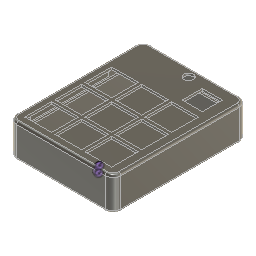
macropad (Autodesk Fusion 360 design; units mm, degrees)
part number: 2026-07-30-09-30-28-857
Autodesk Fusion 360 part; units mm, degrees
note: some values were not read from the file. Set by a fixed rule: which sketch regions a step uses.
(part 1 of 2)
sketch "Sketch1" plane through (0, 0, 0) normal (0, 0, 1) x (1, 0, 0)
  line L0 (0, 0) -> (61.8, 0)
  line L1 (61.8, 0) -> (61.8, 80.8)
  line L2 (61.8, 80.8) -> (0, 80.8)
  line L3 (0, 80.8) -> (0, 0)
  line L4 (-2.3, 78.1) -> (-2.3, 2.7)
  line L5 (2.7, -2.3) -> (59.1, -2.3)
  line L6 (64.1, 2.7) -> (64.1, 78.1)
  line L7 (59.1, 83.1) -> (2.7, 83.1)
  arc A0 (2.7, 83.1) -> (-2.3, 78.1) centre (2.7, 78.1) ccw
  arc A1 (64.1, 78.1) -> (59.1, 83.1) centre (59.1, 78.1) ccw
  arc A2 (59.1, -2.3) -> (64.1, 2.7) centre (59.1, 2.7) ccw
  arc A3 (-2.3, 2.7) -> (2.7, -2.3) centre (2.7, 2.7) ccw
  line L8 (60.5, 1.3) -> (60.5, 79.5)
  line L9 (60.5, 79.5) -> (1.3, 79.5)
  line L10 (1.3, 79.5) -> (1.3, 1.3)
  line L11 (1.3, 1.3) -> (60.5, 1.3)
  dimension "d1" = 61.8
  dimension "d2" = 80.8
  dimension "d4" = 5
  dimension "d5" = 5
  dimension "d6" = 5
  dimension "d7" = 5
  dimension "d17" = -1.3
  constraint horizontal L0
  constraint vertical L1
  constraint horizontal L2
  constraint vertical L3
  constraint coincident L0.start L3.end
  constraint tangent L4 A0
  constraint tangent L7 A0
  constraint tangent L6 A1
  constraint tangent L7 A1
  constraint tangent L5 A2
  constraint tangent L6 A2
  constraint tangent L4 A3
  constraint tangent L5 A3
  measures "d1" distance of L0.start L0.end
  measures "d2" distance of L0.start L2.end
  measures "d4" radius of A0
  measures "d5" radius of A1
  measures "d6" radius of A2
  measures "d7" radius of A3
extrude "Extrude1" add sketch "Sketch1" along normal blind 13.5 contours L0 L1 L2 L3 picked at (0.433333, 53.433333) makes body 1
extrude "Extrude2" add sketch "Sketch1" along normal blind 19.8 contours L4 L5 L6 L7 A0 A1 A2 A3 picked at (-0.766667, 52.966667) bodies 1
sketch "Sketch2" plane through (-2.3, 0, 0) normal (-1, 0, 0) x (0, -1, 0)
  line L0 (-78.1, 0) -> (-2.7, 0)
  line L1 (-2.7, 0) -> (-2.7, 19.8)
  line L2 (-2.7, 19.8) -> (-78.1, 19.8)
  line L3 (-78.1, 19.8) -> (-78.1, 0)
  line L4 (-74, 19.8) -> (-65, 19.8)
  line L5 (-65, 19.8) -> (-65, 16.2)
  line L6 (-65, 16.2) -> (-74, 16.2)
  line L7 (-74, 16.2) -> (-74, 19.8)
  line L8 (-78.1, 0) -> (-2.7, 0)
  point P0 (-80.8, 19.8)
  point P1 (-83.1, 19.8)
  dimension "d12" = 9
  dimension "d13" = 3.6
  dimension "d24" = 6.8
  constraint horizontal L4
  constraint vertical L5
  constraint horizontal L6
  constraint vertical L7
  constraint horizontal L4.start P1
  measures "d12" distance of L4.start L4.end
  measures "d13" distance of L4.start L6.end
  measures "d24" distance of L7 P0
extrude "Extrude3" add sketch "Sketch1" along normal blind 1.5 contours L8 L9 L10 L11 picked at (21.033333, 27.366667) bodies 1
extrude "Extrude4" cut sketch "Sketch2" against normal blind 13 contours L2 L4 L5 L6 L7 picked at (-71, 18.6) bodies 1
fillet "Fillet1" radius 0.5 2 edges at (-1.15, 74, 16.2) (-1.15, 65, 16.2) on bodies 1
sketch "Sketch4" plane through (0, 0, 0) normal (0, 0, 1) x (1, 0, 0)
  line L0 (97.7, 78.1) -> (97.7, 2.7)
  line L1 (100, 0) -> (161.8, 0)
  arc A0 (164.1, 78.1) -> (159.1, 83.1) centre (159.1, 78.1) ccw
  line L2 (161.8, 80.8) -> (100, 80.8)
  arc A1 (97.7, 2.7) -> (102.7, -2.3) centre (102.7, 2.7) ccw
  arc A2 (159.1, -2.3) -> (164.1, 2.7) centre (159.1, 2.7) ccw
  line L3 (102.7, -2.3) -> (159.1, -2.3)
  line L4 (164.1, 2.7) -> (164.1, 78.1)
  line L5 (161.8, 0) -> (161.8, 80.8)
  line L6 (100, 80.8) -> (100, 0)
  arc A3 (102.7, 83.1) -> (97.7, 78.1) centre (102.7, 78.1) ccw
  line L7 (159.1, 83.1) -> (102.7, 83.1)
  line L8 (160.4, 67.5) -> (162.4, 67.5)
  line L9 (162.4, 67.5) -> (162.4, 7.5)
  line L10 (162.4, 7.5) -> (160.4, 7.5)
  line L11 (160.4, 7.5) -> (160.4, 67.5)
  line L12 (161.8, 40.4) -> (175, 40.4) construction
  line L13 (100, 32.5) -> (87.946958, 32.5) construction
  line L14 (99.4, 57.5) -> (101.4, 57.5)
  line L15 (101.4, 57.5) -> (101.4, 7.5)
  line L16 (101.4, 7.5) -> (99.4, 7.5)
  line L17 (99.4, 7.5) -> (99.4, 57.5)
  line L18 (137.8, 79.4) -> (157.8, 79.4)
  line L19 (157.8, 79.4) -> (157.8, 81.4)
  line L20 (157.8, 81.4) -> (137.8, 81.4)
  line L21 (137.8, 81.4) -> (137.8, 79.4)
  line L22 (110.9, -0.6) -> (150.9, -0.6)
  line L23 (150.9, -0.6) -> (150.9, 1.4)
  line L24 (150.9, 1.4) -> (110.9, 1.4)
  line L25 (110.9, 1.4) -> (110.9, -0.6)
  line L26 (130.9, 0) -> (130.9, -7) construction
  point P0 (100, 0)
  dimension "d26" = 61.8
  dimension "d27" = 80.8
  dimension "d28" = 2.3
  dimension "d30" = 2.3
  dimension "d31" = 2.3
  dimension "d32" = 5
  dimension "d33" = 5
  dimension "d34" = 5
  dimension "d35" = 5
  dimension "d36" = 2
  dimension "d37" = 60
  dimension "d38" = 1.4
  dimension "d39" = 32.5
  dimension "d40" = 2
  dimension "d41" = 50
  dimension "d42" = 1.4
  dimension "d123" = 20
  dimension "d124" = 2
  dimension "d125" = 1.4
  dimension "d126" = 40
  dimension "d127" = 2
  dimension "d128" = 1.4
  dimension "d131" = 4
  dimension "d153" = 2.3
  constraint horizontal L1
  constraint vertical L5
  constraint horizontal L2
  constraint vertical L6
  constraint coincident P0 L1.start
  constraint tangent L0 A3
  constraint tangent A3 L7
  constraint tangent A0 L4
  constraint tangent A0 L7
  constraint tangent A2 L3
  constraint tangent A2 L4
  constraint tangent L0 A1
  constraint tangent A1 L3
  constraint horizontal L8
  constraint vertical L9
  constraint horizontal L10
  constraint vertical L11
  constraint midpoint L5 L12.start
  constraint perpendicular L4 L12
  constraint coincident L6 L13.start
  constraint perpendicular L6 L13
  constraint horizontal L14
  constraint vertical L15
  constraint horizontal L16
  constraint vertical L17
  constraint symmetric L13 L14 L16
  constraint horizontal L10.end L15.end
  constraint horizontal L18
  constraint vertical L19
  constraint horizontal L20
  constraint vertical L21
  constraint horizontal L22
  constraint vertical L23
  constraint horizontal L24
  constraint vertical L25
  constraint midpoint L1 L26.start
  constraint perpendicular L3 L26
  constraint symmetric L23 L25 L26
  measures "d26" distance of P0 L1.end
  measures "d27" distance of L2.end P0
  measures "d28" distance of L0 L6
  measures "d30" distance of L4 L5
  measures "d31" distance of L2 L7
  measures "d32" radius of A3
  measures "d33" radius of A0
  measures "d34" radius of A2
  measures "d35" radius of A1
  measures "d36" distance of L8.start L8.end
  measures "d37" distance of L8.start L10.end
  measures "d38" distance of L5 L11
  measures "d39" distance of L1 L13
  measures "d40" distance of L14.start L14.end
  measures "d41" distance of L14.start L16.end
  measures "d42" distance of L6 L15
  measures "d123" distance of L18.start L18.end
  measures "d124" distance of L18.start L20.end
  measures "d125" distance of L2 L18
  measures "d126" distance of L22.start L22.end
  measures "d127" distance of L22.start L24.end
  measures "d128" distance of L1 L24
  measures "d131" distance of L5 L19
  measures "d153" distance of L1 L3
extrude "Extrude5" add sketch "Sketch4" against normal blind 1.5 separate body contours L0 A0 A1 A2 L3 L4 A3 L7 | L1 L2 L5 L6 L8 L10 L11 L14 L15 L16 L18 L19 L21 L23 L24 L25 | L1 L23 L24 L25 | L1 L22 L23 L25 | L6 L14 L16 L17 | L6 L14 L15 L16 | L5 L8 L10 L11 | L5 L8 L9 L10 | L2 L19 L20 L21 | L2 L18 L19 L21 picked at (113.5, 81.566667) picked at (140.733333, 44.166667) picked at (124.233333, 0.933333) picked at (124.233333, -0.4) picked at (99.6, 40.833333) picked at (100.466667, 24.166667) picked at (161.333333, 27.5) picked at (162, 47.5) picked at (144.466667, 81.2) picked at (144.466667, 79.866667) makes body 2
extrude "Extrude6" add sketch "Sketch4" against normal blind 5.5 contours L1 L23 L24 L25 | L1 L22 L23 L25 | L6 L14 L16 L17 | L6 L14 L15 L16 | L5 L8 L10 L11 | L5 L8 L9 L10 | L2 L19 L20 L21 | L2 L18 L19 L21 picked at (124.233333, 0.933333) picked at (124.233333, -0.4) picked at (99.6, 40.833333) picked at (100.466667, 24.166667) picked at (161.333333, 27.5) picked at (162, 47.5) picked at (144.466667, 81.2) picked at (144.466667, 79.866667) bodies 2
sketch "Sketch5" plane through (0, 7.5, 0) normal (0, -1, 0) x (1, 0, 0)
  line L0 (101.4, -1.5) -> (99.4, -1.5)
  line L1 (99.4, -1.5) -> (99.4, -5.5)
  line L2 (99.4, -5.5) -> (101.4, -5.5)
  line L3 (101.40018, -1.5) -> (101.90018, -1.500023)
  line L4 (101.4, -5.5) -> (101.90018, -1.500023)
  line L5 (101.40018, -1.5) -> (99.4, -1.5)
  line L6 (99.4, -5.5) -> (99.4, -1.5)
  line L7 (99.4, -5.5) -> (101.4, -5.5)
  line L8 (100.599998, -1.5) -> (100.599998, -5.5)
  line L9 (100.599998, -5.5) -> (99.6, -3.447432)
  line L10 (99.6, -3.447432) -> (100.599998, -1.5)
  line L11 (159.1, -1.5) -> (102.7, -1.5) construction
  line L12 (130.9, -1.5) -> (130.9, -4) construction
  line L13 (160.39982, -1.5) -> (162.4, -1.5)
  line L14 (160.4, -1.5) -> (162.4, -1.5)
  line L15 (162.4, -5.5) -> (162.4, -1.5)
  line L16 (161.200002, -5.5) -> (162.2, -3.447432)
  line L17 (162.2, -3.447432) -> (161.200002, -1.5)
  line L18 (160.4, -5.5) -> (159.89982, -1.500023)
  line L19 (162.4, -5.5) -> (160.4, -5.5)
  line L20 (160.39982, -1.5) -> (159.89982, -1.500023)
  line L21 (161.200002, -1.5) -> (161.200002, -5.5)
  line L22 (162.4, -5.5) -> (160.4, -5.5)
  line L23 (162.4, -1.5) -> (162.4, -5.5)
  point P0 (102.8, -1.5)
  point P1 (159.1, -1.5)
  point P2 (159, -1.5)
  dimension "d58" = 0.5
  dimension "d65" = 0.2
  dimension "d66" = 1
  constraint coincident L2.end L4.start
  constraint coincident L0.end L1.start
  constraint perpendicular L1 L5
  constraint coincident L1.end L2.start
  constraint perpendicular L7 L8
  constraint midpoint L11 L12.start
  constraint perpendicular L11 L12
  constraint symmetric L0.start L12 L14.start
  constraint symmetric L0.end L12 L13.end
  constraint symmetric L1.end L12 L15.start
  constraint symmetric L2.end L12 L18.start
  constraint symmetric P0 L12 P2
  constraint symmetric L11.end L12 P1
extrude "Extrude7" cut sketch "Sketch5" against normal blind 69 contours L0 L1 L2 L5 L6 L7 L9 L10 | L13 L14 L15 L16 L17 L19 L22 L23 picked at (99.866666, -4.815811) picked at (161.933334, -4.815811) bodies 2
extrude "Extrude8" add sketch "Sketch5" against normal blind 50 contours L0 L2 L3 L4 L5 L7 L8 picked at (100.866665, -2.833333) bodies 2
extrude "Extrude9" add sketch "Sketch5" against normal blind 60 contours L13 L14 L18 L19 L20 L21 L22 picked at (160.666607, -2.833333) bodies 2
sketch "Sketch8" plane through (150.9, 0, 0) normal (1, 0, 0) x (0, 1, 0)
  line L0 (1.4, -1.5) -> (-0.6, -1.5)
  line L1 (-0.6, -1.5) -> (-0.6, -5.5)
  line L2 (-0.6, -5.5) -> (1.4, -5.5)
  line L3 (1.4, -5.5) -> (1.4, -1.5)
  line L4 (1.40018, -1.5) -> (-0.6, -1.5)
  line L5 (1.4, -1.5) -> (-0.6, -1.5)
  line L6 (-0.6, -5.5) -> (1.4, -5.5)
  line L7 (-0.4, -3.447432) -> (0.599998, -1.5)
  line L8 (0.599998, -5.5) -> (-0.4, -3.447432)
  line L9 (-0.6, -1.5) -> (-0.6, -5.5)
  line L10 (0.599998, -1.5) -> (0.599998, -5.5)
  line L11 (-0.6, -5.5) -> (-0.6, -1.5)
  line L12 (1.40018, -1.5) -> (1.90018, -1.500023)
  line L13 (1.4, -5.5) -> (1.90018, -1.500023)
  line L14 (-0.6, -5.5) -> (1.4, -5.5)
  line L15 (78.1, -1.5) -> (2.7, -1.5) construction
  line L16 (40.4, -1.5) -> (40.4, -9) construction
  line L17 (81.4, -5.5) -> (79.4, -5.5)
  line L18 (81.2, -3.447432) -> (80.200002, -1.5)
  line L19 (79.4, -1.5) -> (81.4, -1.5)
  line L20 (79.39982, -1.5) -> (78.89982, -1.500023)
  line L21 (81.4, -5.5) -> (81.4, -1.5)
  line L22 (81.4, -5.5) -> (79.4, -5.5)
  line L23 (79.39982, -1.5) -> (81.4, -1.5)
  line L24 (81.4, -1.5) -> (81.4, -5.5)
  line L25 (79.4, -5.5) -> (79.4, -1.5)
  line L26 (80.200002, -5.5) -> (81.2, -3.447432)
  line L27 (81.4, -1.5) -> (81.4, -5.5)
  line L28 (79.4, -5.5) -> (78.89982, -1.500023)
  line L29 (80.200002, -1.5) -> (80.200002, -5.5)
  line L30 (79.4, -1.5) -> (81.4, -1.5)
  line L31 (81.4, -5.5) -> (79.4, -5.5)
  point P0 (2.8, -1.5)
  dimension "d132" = 0.5
  dimension "d133" = 0.2
  dimension "d134" = 1
  constraint coincident L2.end L3.start
  constraint coincident L0.end L1.start
  constraint perpendicular L4 L9
  constraint coincident L1.end L2.start
  constraint perpendicular L6 L10
  constraint midpoint L15 L16.start
  constraint perpendicular L15 L16
  constraint symmetric L0.start L16 L19.start
  constraint symmetric L0.end L16 L19.end
  constraint symmetric L1.end L16 L17.start
  constraint symmetric L2.end L16 L17.end
extrude "Extrude13" cut sketch "Sketch8" along normal blind 13 and the other way blind 46.5 contours L0 L1 L2 L4 L5 L6 L7 L8 L9 L11 L14 | L17 L18 L19 L21 L22 L23 L24 L26 L27 L30 L31 picked at (-0.133334, -4.815811) picked at (80.933334, -4.815811) bodies 2
extrude "Extrude14" add sketch "Sketch8" against normal blind 40 contours L3 L12 L13 picked at (1.566727, -2.833341) bodies 2
extrude "Extrude15" add sketch "Sketch8" along normal blind 6.9 and the other way blind 13.1 contours L20 L25 L28 picked at (79.233273, -2.833341) bodies 2
move_body "Move1" bodies 2 to x (1, 0, 0) y (0, 1, 0) z (0, 0, 1) at (-100, 0, 21.3)
ref_plane "WorkPlane1" through (30.9, 7.7, 9.9) normal (0, -1, 0) x (1, 0, 0)
sketch "Sketch6" plane through (0, 7.7, 0) normal (0, -1, 0) x (-1, 0, 0)
  line L0 (-0.599998, -15.8) -> (-1.4, -15.8)
  line L1 (-1.40018, -19.8) -> (-0.599998, -19.8)
  line L2 (-61.200002, -19.8) -> (-60.39982, -19.8)
  line L3 (-60.4, -15.8) -> (-61.200002, -15.8)
  line L4 (-0.599998, -19.8) -> (0.4, -17.852568)
  line L5 (0.4, -17.852568) -> (-0.599998, -15.8)
  line L6 (-1.4, -15.8) -> (-1.90018, -19.799977)
  line L7 (-1.90018, -19.799977) -> (-1.40018, -19.8)
  line L8 (-60.39982, -19.8) -> (-59.89982, -19.799977)
  line L9 (-59.89982, -19.799977) -> (-60.4, -15.8)
  line L10 (-61.200002, -15.8) -> (-62.2, -17.852568)
  line L11 (-62.2, -17.852568) -> (-61.200002, -19.8)
extrude "Extrude10" cut sketch "Sketch6" against normal blind 50 contours L0 L1 L4 L5 L6 L7 picked at (-0.80006, -17.817523) bodies 1
extrude "Extrude11" cut sketch "Sketch6" against normal blind 60 contours L2 L3 L8 L9 L10 L11 picked at (-60.99994, -17.817523) bodies 1
sketch "Sketch7" plane through (0, 0, 21.3) normal (0, 0, 1) x (-1, 0, 0)
  line L0 (-59.1, -83.1) -> (-2.7, -83.1)
  arc A0 (-2.7, -83.1) -> (2.3, -78.1) centre (-2.7, -78.1) ccw
  line L1 (2.3, -78.1) -> (2.3, -2.7)
  arc A1 (2.3, -2.7) -> (-2.7, 2.3) centre (-2.7, -2.7) ccw
  line L2 (-2.7, 2.3) -> (-59.1, 2.3)
  arc A2 (-59.1, 2.3) -> (-64.1, -2.7) centre (-59.1, -2.7) ccw
  line L3 (-64.1, -2.7) -> (-64.1, -78.1)
  arc A3 (-64.1, -78.1) -> (-59.1, -83.1) centre (-59.1, -78.1) ccw
  circle A4 centre (-49.8, -68.8) radius 4
  line L4 (-43.8, -74.8) -> (-55.8, -74.8)
  line L5 (-55.8, -74.8) -> (-55.8, -62.8)
  line L6 (-55.8, -62.8) -> (-43.8, -62.8)
  line L7 (-43.8, -62.8) -> (-43.8, -74.8)
  line L8 (2.3, -74) -> (0, -74)
  line L9 (0, -74) -> (0, -80.8)
  line L10 (0, -80.8) -> (-61.8, -80.8)
  line L11 (-61.8, -80.8) -> (-61.8, 0)
  line L12 (-61.8, 0) -> (0, 0)
  line L13 (0, 0) -> (0, -65)
  line L14 (0, -65) -> (2.3, -65)
  line L15 (2.3, -65) -> (2.3, -2.7)
  arc A5 (2.3, -2.7) -> (-2.7, 2.3) centre (-2.7, -2.7) ccw
  line L16 (-2.7, 2.3) -> (-59.1, 2.3)
  arc A6 (-59.1, 2.3) -> (-64.1, -2.7) centre (-59.1, -2.7) ccw
  line L17 (-64.1, -2.7) -> (-64.1, -78.1)
  arc A7 (-64.1, -78.1) -> (-59.1, -83.1) centre (-59.1, -78.1) ccw
  line L18 (-59.1, -83.1) -> (-2.7, -83.1)
  arc A8 (-2.7, -83.1) -> (2.3, -78.1) centre (-2.7, -78.1) ccw
  line L19 (2.3, -78.1) -> (2.3, -74)
  circle A9 centre (-32.7, -77.3) radius 3
  line L20 (-3.4, -19.3) -> (-19, -19.3)
  line L21 (-19, -19.3) -> (-19, -3.7)
  line L22 (-19, -3.7) -> (-3.4, -3.7)
  line L23 (-3.4, -3.7) -> (-3.4, -19.3)
  line L24 (-22.5, -19.3) -> (-38.1, -19.3)
  line L25 (-38.1, -19.3) -> (-38.1, -3.7)
  line L26 (-38.1, -3.7) -> (-22.5, -3.7)
  line L27 (-22.5, -3.7) -> (-22.5, -19.3)
  line L28 (-41.6, -19.3) -> (-57.2, -19.3)
  line L29 (-57.2, -19.3) -> (-57.2, -3.7)
  line L30 (-57.2, -3.7) -> (-41.6, -3.7)
  line L31 (-41.6, -3.7) -> (-41.6, -19.3)
  line L32 (-3.4, -38.4) -> (-19, -38.4)
  line L33 (-19, -38.4) -> (-19, -22.8)
  line L34 (-19, -22.8) -> (-3.4, -22.8)
  line L35 (-3.4, -22.8) -> (-3.4, -38.4)
  line L36 (-22.5, -41.9) -> (-22.5, -57.5)
  line L37 (-38.1, -41.9) -> (-22.5, -41.9)
  line L38 (-38.1, -57.5) -> (-38.1, -41.9)
  line L39 (-22.5, -57.5) -> (-38.1, -57.5)
  line L40 (-3.4, -41.9) -> (-3.4, -57.5)
  line L41 (-19, -41.9) -> (-3.4, -41.9)
  line L42 (-19, -57.5) -> (-19, -41.9)
  line L43 (-3.4, -57.5) -> (-19, -57.5)
  line L44 (-22.5, -22.8) -> (-22.5, -38.4)
  line L45 (-38.1, -22.8) -> (-22.5, -22.8)
  line L46 (-38.1, -38.4) -> (-38.1, -22.8)
  line L47 (-22.5, -38.4) -> (-38.1, -38.4)
  line L48 (-41.6, -22.8) -> (-41.6, -38.4)
  line L49 (-57.2, -22.8) -> (-41.6, -22.8)
  line L50 (-57.2, -38.4) -> (-57.2, -22.8)
  line L51 (-41.6, -38.4) -> (-57.2, -38.4)
  line L52 (-41.6, -41.9) -> (-41.6, -57.5)
  line L53 (-57.2, -41.9) -> (-41.6, -41.9)
  line L54 (-57.2, -57.5) -> (-57.2, -41.9)
  line L55 (-41.6, -57.5) -> (-57.2, -57.5)
  line L56 (-19.7, -41.2) -> (-2.7, -41.2)
  line L57 (-2.7, -41.2) -> (-2.7, -58.2)
  line L58 (-2.7, -58.2) -> (-19.7, -58.2)
  line L59 (-19.7, -58.2) -> (-19.7, -41.2)
  line L60 (-38.8, -41.2) -> (-21.8, -41.2)
  line L61 (-21.8, -41.2) -> (-21.8, -58.2)
  line L62 (-21.8, -58.2) -> (-38.8, -58.2)
  line L63 (-38.8, -58.2) -> (-38.8, -41.2)
  line L64 (-57.9, -41.2) -> (-40.9, -41.2)
  line L65 (-40.9, -41.2) -> (-40.9, -58.2)
  line L66 (-40.9, -58.2) -> (-57.9, -58.2)
  line L67 (-57.9, -58.2) -> (-57.9, -41.2)
  line L68 (-19.7, -22.1) -> (-2.7, -22.1)
  line L69 (-2.7, -22.1) -> (-2.7, -39.1)
  line L70 (-2.7, -39.1) -> (-19.7, -39.1)
  line L71 (-19.7, -39.1) -> (-19.7, -22.1)
  line L72 (-38.8, -22.1) -> (-21.8, -22.1)
  line L73 (-21.8, -22.1) -> (-21.8, -39.1)
  line L74 (-21.8, -39.1) -> (-38.8, -39.1)
  line L75 (-38.8, -39.1) -> (-38.8, -22.1)
  line L76 (-57.9, -22.1) -> (-40.9, -22.1)
  line L77 (-40.9, -22.1) -> (-40.9, -39.1)
  line L78 (-40.9, -39.1) -> (-57.9, -39.1)
  line L79 (-57.9, -39.1) -> (-57.9, -22.1)
  line L80 (-19.7, -3) -> (-2.7, -3)
  line L81 (-2.7, -3) -> (-2.7, -20)
  line L82 (-2.7, -20) -> (-19.7, -20)
  line L83 (-19.7, -20) -> (-19.7, -3)
  line L84 (-38.8, -3) -> (-21.8, -3)
  line L85 (-21.8, -3) -> (-21.8, -20)
  line L86 (-21.8, -20) -> (-38.8, -20)
  line L87 (-38.8, -20) -> (-38.8, -3)
  line L88 (-57.9, -3) -> (-40.9, -3)
  line L89 (-40.9, -3) -> (-40.9, -20)
  line L90 (-40.9, -20) -> (-57.9, -20)
  line L91 (-57.9, -20) -> (-57.9, -3)
  line L92 (-56.2, -75.2) -> (-56.2, -62.4)
  line L93 (-56.2, -62.4) -> (-43.4, -62.4)
  line L94 (-43.4, -62.4) -> (-43.4, -75.2)
  line L95 (-43.4, -75.2) -> (-56.2, -75.2)
  dimension "d70" = 8
  dimension "d73" = 12
  dimension "d74" = 12
  dimension "d75" = 6
  dimension "d76" = 6
  dimension "d79" = 6
  dimension "d80" = 6
  dimension "d81" = 6
  dimension "d83" = 35
  dimension "d84" = 5.8
  dimension "d85" = 15.6
  dimension "d86" = 15.6
  dimension "d87" = 3.7
  dimension "d88" = 3.4
  dimension "d89" = 15.6
  dimension "d90" = 15.6
  dimension "d91" = 3.5
  dimension "d92" = 15.6
  dimension "d93" = 15.6
  dimension "d94" = 3.5
  dimension "d95" = 15.6
  dimension "d96" = 15.6
  dimension "d97" = 15.6
  dimension "d98" = 15.6
  dimension "d99" = 15.6
  dimension "d100" = 15.6
  dimension "d101" = 15.6
  dimension "d102" = 15.6
  dimension "d103" = 15.6
  dimension "d104" = 15.6
  dimension "d105" = 15.6
  dimension "d106" = 15.6
  dimension "d107" = 3.5
  dimension "d108" = 3.5
  dimension "d109" = -0.7
  dimension "d110" = -0.7
  dimension "d111" = -0.7
  dimension "d112" = -0.7
  dimension "d113" = -0.7
  dimension "d114" = -0.7
  dimension "d115" = -0.7
  dimension "d116" = -0.7
  dimension "d117" = -0.7
  dimension "d121" = -0.4
  constraint horizontal L4
  constraint vertical L5
  constraint horizontal L6
  constraint vertical L7
  constraint horizontal L20
  constraint vertical L21
  constraint horizontal L22
  constraint vertical L23
  constraint horizontal L24
  constraint vertical L25
  constraint horizontal L26
  constraint vertical L27
  constraint horizontal L20.end L24.start
  constraint horizontal L28
  constraint vertical L29
  constraint horizontal L30
  constraint vertical L31
  constraint horizontal L24.end L28.start
  constraint horizontal L32
  constraint perpendicular L32 L33
  constraint perpendicular L33 L34
  constraint perpendicular L32 L35
  constraint horizontal L39
  constraint perpendicular L38 L39
  constraint perpendicular L37 L38
  constraint perpendicular L36 L39
  constraint horizontal L43
  constraint perpendicular L42 L43
  constraint perpendicular L41 L42
  constraint perpendicular L40 L43
  constraint horizontal L47
  constraint perpendicular L46 L47
  constraint perpendicular L45 L46
  constraint perpendicular L44 L47
  constraint horizontal L51
  constraint perpendicular L50 L51
  constraint perpendicular L49 L50
  constraint perpendicular L48 L51
  constraint horizontal L55
  constraint perpendicular L54 L55
  constraint perpendicular L53 L54
  constraint perpendicular L52 L55
  constraint vertical L20.start L34.end
  constraint vertical L32.start L40.start
  constraint horizontal L36.end L42.start
  constraint vertical L24.start L36.end
  constraint horizontal L32.end L44.end
  constraint vertical L24.start L44.end
  constraint horizontal L38.start L52.end
  constraint vertical L28.start L52.end
  constraint horizontal L46.start L48.end
  constraint vertical L28.start L48.end
  measures "d70" diameter of A4
  measures "d73" distance of L4.start L4.end
  measures "d74" distance of L4.start L6.end
  measures "d75" distance of A4.centre L4
  measures "d76" distance of A4.centre L5
  measures "d79" distance of L4 L10
  measures "d80" distance of L5 L11
  measures "d81" diameter of A9
  measures "d83" distance of L19 A9.centre
  measures "d84" distance of L18 A9.centre
  measures "d85" distance of L20.start L20.end
  measures "d86" distance of L20.start L22.end
  measures "d87" distance of L12 L22
  measures "d88" distance of L13 L23
  measures "d89" distance of L24.start L24.end
  measures "d90" distance of L24.start L26.end
  measures "d91" distance of L21 L27
  measures "d92" distance of L28.start L28.end
  measures "d93" distance of L28.start L30.end
  measures "d94" distance of L25 L31
  measures "d95" distance of L32.start L32.end
  measures "d96" distance of L32 L34
  measures "d97" distance of L36.end L38.start
  measures "d98" distance of L37 L39
  measures "d99" distance of L40.end L42.start
  measures "d100" distance of L41 L43
  measures "d101" distance of L44.end L46.start
  measures "d102" distance of L45 L47
  measures "d103" distance of L48.end L50.start
  measures "d104" distance of L49 L51
  measures "d105" distance of L52.end L54.start
  measures "d106" distance of L53 L55
  measures "d107" distance of L20 L34
  measures "d108" distance of L32 L41
extrude "Extrude12" cut sketch "Sketch7" against normal blind 9 contours A4 | L4 L5 L6 L7 | A9 | L20 L21 L22 L23 | L24 L25 L26 L27 | L28 L29 L30 L31 | L32 L33 L34 L35 | L36 L37 L38 L39 | L40 L41 L42 L43 | L44 L45 L46 L47 | L48 L49 L50 L51 | L52 L53 L54 L55 | L56 L57 L58 L59 | L60 L61 L62 L63 | L64 L65 L66 L67 | L68 L69 L70 L71 | L72 L73 L74 L75 | L76 L77 L78 L79 | L80 L81 L82 L83 | L84 L85 L86 L87 | L88 L89 L90 L91 | L92 L93 L94 L95 picked at (-49.312879, -70.438611) picked at (-49.70036, -74.129605) picked at (-31.013745, -77.005245) picked at (-13.8, -14.1) picked at (-27.7, -14.1) picked at (-46.8, -8.9) picked at (-8.6, -33.2) picked at (-32.9, -47.1) picked at (-8.6, -52.3) picked at (-32.9, -28) picked at (-52, -28) picked at (-52, -47.1) picked at (-13.8, -57.966667) picked at (-38.566667, -52.3) picked at (-52, -41.433333) picked at (-8.6, -38.866667) picked at (-27.7, -38.866667) picked at (-57.666667, -33.2) picked at (-8.6, -19.766667) picked at (-27.7, -19.766667) picked at (-41.133333, -14.1) picked at (-56.066667, -66.8) bodies 2
ref_plane "WorkPlane2" through (51.7, 40.4, 9.9) normal (1, 0, 0) x (0, 1, 0)
sketch "Sketch9" plane through (51.7, 0, 0) normal (1, 0, 0) x (0, 1, 0)
  line L0 (0.599998, 15.8) -> (-0.4, 17.852568)
  line L1 (-0.4, 17.852568) -> (0.599998, 19.8)
  line L2 (0.599998, 19.8) -> (1.40018, 19.8)
  line L3 (1.40018, 19.8) -> (1.90018, 19.799977)
  line L4 (1.90018, 19.799977) -> (1.4, 15.8)
  line L5 (1.4, 15.8) -> (0.599998, 15.8)
extrude "Extrude16" cut sketch "Sketch9" against normal blind 40 bodies 1
ref_plane "WorkPlane3" through (58.6001, 40.4, 9.9) normal (1, 0, 0) x (0, 1, 0)
sketch "Sketch10" plane through (58.6001, 0, 0) normal (1, 0, 0) x (0, 1, 0)
  line L0 (80.200002, 15.8) -> (81.2, 17.852568)
  line L1 (81.2, 17.852568) -> (80.200002, 19.8)
  line L2 (80.200002, 19.8) -> (79.39982, 19.8)
  line L3 (79.39982, 19.8) -> (78.89982, 19.799977)
  line L4 (78.89982, 19.799977) -> (79.4, 15.8)
  line L5 (79.4, 15.8) -> (80.200002, 15.8)
extrude "Extrude17" cut sketch "Sketch10" against normal blind 20 bodies 1
sketch "Sketch11" plane through (0, 0, 0) normal (0, 0, -1) x (1, 0, 0)
  arc A0 (2.7, 2.3) -> (-2.3, -2.7) centre (2.7, -2.7) ccw
  line L0 (-2.3, -2.7) -> (-2.3, -78.1)
  arc A1 (-2.3, -78.1) -> (2.7, -83.1) centre (2.7, -78.1) ccw
  line L1 (2.7, -83.1) -> (59.1, -83.1)
  arc A2 (59.1, -83.1) -> (64.1, -78.1) centre (59.1, -78.1) ccw
  line L2 (64.1, -78.1) -> (64.1, -2.7)
  arc A3 (64.1, -2.7) -> (59.1, 2.3) centre (59.1, -2.7) ccw
  line L3 (59.1, 2.3) -> (2.7, 2.3)
  spline S0 degree 3 poles (2.059624, -40.593318) (0.638908, -39.614032) (-0.26253, -37.866887) (0.339903, -36.133014) knots 0 0 0 0 1 1 1 1
  spline S1 degree 3 poles (0.339903, -36.133014) (0.608829, -35.359848) (1.252842, -34.893646) (1.773891, -34.312443) knots 0 0 0 0 1 1 1 1
  spline S2 degree 3 poles (1.773891, -34.312443) (1.611116, -33.06246) (1.521768, -31.316201) (1.642082, -30.068874) knots 0 0 0 0 1 1 1 1
  spline S3 degree 3 poles (1.642082, -30.068874) (1.691621, -29.562863) (1.797772, -29.061279) (1.867661, -28.55969) knots 0 0 0 0 1 1 1 1
  spline S4 degree 3 poles (1.867661, -28.55969) (1.94816, -27.9838) (1.798657, -27.316785) (2.03043, -26.766548) knots 0 0 0 0 1 1 1 1
  spline S5 degree 3 poles (2.03043, -26.766548) (2.723097, -25.124674) (5.522069, -24.129465) (7.146248, -23.998536) knots 0 0 0 0 1 1 1 1
  spline S6 degree 3 poles (7.146248, -23.998536) (7.559369, -23.964925) (7.965417, -23.8915) (8.382074, -23.937497) knots 0 0 0 0 1 1 1 1
  spline S7 degree 3 poles (8.382074, -23.937497) (9.120744, -24.020652) (9.746178, -24.320543) (10.419381, -24.600089) knots 0 0 0 0 1 1 1 1
  spline S8 degree 3 poles (10.419381, -24.600089) (11.057201, -24.080812) (11.73394, -23.539413) (12.42307, -23.089139) knots 0 0 0 0 1 1 1 1
  spline S9 degree 3 poles (12.42307, -23.089139) (12.87423, -22.79367) (13.361662, -22.561012) (13.8199, -22.276164) knots 0 0 0 0 1 1 1 1
  spline S10 degree 3 poles (13.8199, -22.276164) (14.34537, -21.950621) (14.847839, -21.57996) (15.386582, -21.275647) knots 0 0 0 0 1 1 1 1
  spline S11 degree 3 poles (15.386582, -21.275647) (15.69266, -21.104029) (16.02086, -20.975756) (16.324288, -20.797059) knots 0 0 0 0 1 1 1 1
  spline S12 degree 3 poles (16.324288, -20.797059) (18.768521, -19.360421) (21.318027, -18.136981) (23.895841, -16.961304) knots 0 0 0 0 1 1 1 1
  spline S13 degree 3 poles (23.895841, -16.961304) (25.218358, -16.357985) (26.529381, -15.734322) (27.881099, -15.197351) knots 0 0 0 0 1 1 1 1
  spline S14 degree 3 poles (27.881099, -15.197351) (28.421607, -14.982386) (29.032884, -14.575458) (29.615857, -14.51707) knots 0 0 0 0 1 1 1 1
  spline S15 degree 3 poles (29.615857, -14.51707) (30.085596, -14.470187) (30.571257, -14.559536) (31.031266, -14.628534) knots 0 0 0 0 1 1 1 1
  spline S16 degree 3 poles (31.031266, -14.628534) (31.616891, -14.716112) (32.214016, -14.72319) (32.79787, -14.818732) knots 0 0 0 0 1 1 1 1
  spline S17 degree 3 poles (32.79787, -14.818732) (33.305652, -14.901887) (33.795736, -15.078813) (34.307054, -15.146926) knots 0 0 0 0 1 1 1 1
  spline S18 degree 3 poles (34.307054, -15.146926) (35.249182, -15.271662) (36.185123, -15.388434) (37.122829, -15.543244) knots 0 0 0 0 1 1 1 1
  spline S19 degree 3 poles (37.122829, -15.543244) (38.043729, -15.695398) (38.982323, -15.956365) (39.874029, -16.232369) knots 0 0 0 0 1 1 1 1
  spline S20 degree 3 poles (39.874029, -16.232369) (40.334038, -16.374793) (40.805545, -16.470335) (41.265554, -16.609223) knots 0 0 0 0 1 1 1 1
  spline S21 degree 3 poles (41.265554, -16.609223) (43.322319, -17.230235) (45.310969, -18.080363) (47.296962, -18.893339) knots 0 0 0 0 1 1 1 1
  spline S22 degree 3 poles (47.296962, -18.893339) (50.579827, -20.237092) (53.869767, -21.714426) (56.834161, -23.683608) knots 0 0 0 0 1 1 1 1
  spline S23 degree 3 poles (56.834161, -23.683608) (57.597598, -24.190505) (59.432321, -25.191022) (59.78352, -26.036728) knots 0 0 0 0 1 1 1 1
  spline S24 degree 3 poles (59.78352, -26.036728) (59.968407, -26.479929) (59.992292, -27.364559) (60.001138, -27.854642) knots 0 0 0 0 1 1 1 1
  spline S25 degree 3 poles (60.001138, -27.854642) (60.029447, -29.302782) (59.802096, -30.669536) (59.657902, -32.100868) knots 0 0 0 0 1 1 1 1
  spline S26 degree 3 poles (59.657902, -32.100868) (60.196642, -32.38395) (60.751305, -32.484799) (61.183004, -32.958074) knots 0 0 0 0 1 1 1 1
  spline S27 degree 3 poles (61.183004, -32.958074) (62.332139, -34.221324) (62.080019, -36.761985) (61.274121, -38.147313) knots 0 0 0 0 1 1 1 1
  spline S28 degree 3 poles (61.274121, -38.147313) (60.894615, -38.798405) (60.358529, -39.306182) (59.870213, -39.867037) knots 0 0 0 0 1 1 1 1
  spline S29 degree 3 poles (59.870213, -39.867037) (60.247065, -42.061805) (60.015292, -44.363612) (59.5774, -46.525649) knots 0 0 0 0 1 1 1 1
  spline S30 degree 3 poles (59.5774, -46.525649) (59.444706, -47.178506) (59.158085, -48.56826) (58.764425, -49.084001) knots 0 0 0 0 1 1 1 1
  spline S31 degree 3 poles (58.764425, -49.084001) (58.405265, -49.555507) (57.680753, -49.710318) (57.169437, -49.968631) knots 0 0 0 0 1 1 1 1
  spline S32 degree 3 poles (57.169437, -49.968631) (56.588234, -50.262326) (56.05038, -50.630333) (55.469177, -50.92403) knots 0 0 0 0 1 1 1 1
  spline S33 degree 3 poles (55.469177, -50.92403) (54.815434, -51.254881) (54.12277, -51.469848) (53.441603, -51.729044) knots 0 0 0 0 1 1 1 1
  spline S34 degree 3 poles (53.441603, -51.729044) (52.538397, -52.073164) (51.695344, -52.589788) (50.810714, -52.982564) knots 0 0 0 0 1 1 1 1
  spline S35 degree 3 poles (50.810714, -52.982564) (50.044624, -53.322264) (49.249342, -53.589422) (48.482366, -53.932659) knots 0 0 0 0 1 1 1 1
  spline S36 degree 3 poles (48.482366, -53.932659) (46.72726, -54.719979) (45.006656, -55.549763) (43.228549, -56.279583) knots 0 0 0 0 1 1 1 1
  spline S37 degree 3 poles (43.228549, -56.279583) (42.350994, -56.640511) (41.541558, -57.155366) (40.667543, -57.526027) knots 0 0 0 0 1 1 1 1
  spline S38 degree 3 poles (40.667543, -57.526027) (40.225228, -57.713568) (39.323789, -57.931186) (38.989399, -58.236385) knots 0 0 0 0 1 1 1 1
  spline S39 degree 3 poles (38.989399, -58.236385) (38.810705, -58.398271) (38.724896, -58.723817) (38.628471, -58.93701) knots 0 0 0 0 1 1 1 1
  spline S40 degree 3 poles (38.628471, -58.93701) (38.423236, -59.389058) (38.16758, -59.813679) (37.848227, -60.194955) knots 0 0 0 0 1 1 1 1
  spline S41 degree 3 poles (37.848227, -60.194955) (36.430164, -61.880177) (33.549806, -63.744978) (31.382462, -64.159868) knots 0 0 0 0 1 1 1 1
  spline S42 degree 3 poles (31.382462, -64.159868) (30.829568, -64.266025) (30.263407, -64.27664) (29.707857, -64.361564) knots 0 0 0 0 1 1 1 1
  spline S43 degree 3 poles (29.707857, -64.361564) (29.151427, -64.445605) (28.587918, -64.579183) (28.023523, -64.610146) knots 0 0 0 0 1 1 1 1
  spline S44 degree 3 poles (28.023523, -64.610146) (26.484264, -64.69507) (24.36823, -64.268679) (23.00059, -63.530012) knots 0 0 0 0 1 1 1 1
  spline S45 degree 3 poles (23.00059, -63.530012) (21.647106, -62.799308) (20.732402, -61.553748) (19.562918, -60.596578) knots 0 0 0 0 1 1 1 1
  spline S46 degree 3 poles (19.562918, -60.596578) (18.554442, -59.771219) (17.503501, -59.161707) (16.325173, -58.61766) knots 0 0 0 0 1 1 1 1
  spline S47 degree 3 poles (16.325173, -58.61766) (15.452929, -58.215154) (14.556798, -58.007266) (13.60405, -57.907302) knots 0 0 0 0 1 1 1 1
  spline S48 degree 3 poles (13.60405, -57.907302) (12.899882, -57.832993) (12.18687, -57.90907) (11.480937, -57.862185) knots 0 0 0 0 1 1 1 1
  spline S49 degree 3 poles (11.480937, -57.862185) (10.801541, -57.817071) (10.120375, -57.722415) (9.446287, -57.631298) knots 0 0 0 0 1 1 1 1
  spline S50 degree 3 poles (9.446287, -57.631298) (9.070319, -57.580873) (8.679314, -57.581759) (8.306883, -57.511872) knots 0 0 0 0 1 1 1 1
  spline S51 degree 3 poles (8.306883, -57.511872) (5.696338, -57.020903) (2.515211, -55.731996) (1.974698, -52.799448) knots 0 0 0 0 1 1 1 1
  spline S52 degree 3 poles (1.974698, -52.799448) (1.759733, -51.630849) (1.873854, -50.346367) (1.930466, -49.168924) knots 0 0 0 0 1 1 1 1
  spline S53 degree 3 poles (1.930466, -49.168924) (1.980891, -48.143638) (1.971161, -47.104198) (1.960546, -46.078026) knots 0 0 0 0 1 1 1 1
  spline S54 degree 3 poles (1.960546, -46.078026) (1.949931, -45.106701) (1.972047, -44.132725) (1.934894, -43.162285) knots 0 0 0 0 1 1 1 1
  spline S55 degree 3 poles (1.934894, -43.162285) (1.903929, -42.328962) (1.820773, -41.402754) (2.059624, -40.593318) knots 0 0 0 0 1 1 1 1
  spline S56 degree 3 poles (56.341421, -48.466528) (54.945475, -47.426202) (53.566337, -46.324838) (52.071312, -45.425168) knots 0 0 0 0 1 1 1 1
  spline S57 degree 3 poles (52.071312, -45.425168) (50.84787, -44.689155) (49.5855, -44.06726) (48.301904, -43.447136) knots 0 0 0 0 1 1 1 1
  spline S58 degree 3 poles (48.301904, -43.447136) (47.227076, -42.927859) (46.174366, -42.367001) (45.074772, -41.898148) knots 0 0 0 0 1 1 1 1
  spline S59 degree 3 poles (45.074772, -41.898148) (42.655307, -40.8649) (40.104034, -40.035117) (37.582838, -39.30176) knots 0 0 0 0 1 1 1 1
  spline S60 degree 3 poles (37.582838, -39.30176) (36.999867, -39.131907) (36.401856, -38.890405) (35.80473, -38.78779) knots 0 0 0 0 1 1 1 1
  spline S61 degree 3 poles (35.80473, -38.78779) (35.638419, -38.758596) (35.47034, -38.778055) (35.304029, -38.743559) knots 0 0 0 0 1 1 1 1
  spline S62 degree 3 poles (35.304029, -38.743559) (34.815717, -38.643595) (34.342436, -38.457819) (33.851468, -38.35697) knots 0 0 0 0 1 1 1 1
  spline S63 degree 3 poles (33.851468, -38.35697) (33.418882, -38.267627) (32.971259, -38.235776) (32.539559, -38.148199) knots 0 0 0 0 1 1 1 1
  spline S64 degree 3 poles (32.539559, -38.148199) (31.789395, -37.996045) (31.038344, -37.629807) (30.247485, -37.745693) knots 0 0 0 0 1 1 1 1
  spline S65 degree 3 poles (30.247485, -37.745693) (29.423009, -37.866887) (28.612684, -38.358741) (27.876677, -38.724094) knots 0 0 0 0 1 1 1 1
  spline S66 degree 3 poles (27.876677, -38.724094) (27.18401, -39.067331) (26.484264, -39.386681) (25.795139, -39.736997) knots 0 0 0 0 1 1 1 1
  spline S67 degree 3 poles (25.795139, -39.736997) (23.801184, -40.749897) (21.811652, -41.773415) (19.814155, -42.776585) knots 0 0 0 0 1 1 1 1
  spline S68 degree 3 poles (19.814155, -42.776585) (18.589824, -43.39229) (17.40796, -44.135379) (16.15444, -44.690041) knots 0 0 0 0 1 1 1 1
  spline S69 degree 3 poles (16.15444, -44.690041) (14.639068, -45.360592) (13.195351, -46.16295) (11.698558, -46.871539) knots 0 0 0 0 1 1 1 1
  spline S70 degree 3 poles (11.698558, -46.871539) (11.433169, -46.997158) (11.112933, -47.111273) (10.874082, -47.281124) knots 0 0 0 0 1 1 1 1
  spline S71 degree 3 poles (10.874082, -47.281124) (10.681233, -47.41824) (10.560919, -47.628783) (10.313224, -47.690708) knots 0 0 0 0 1 1 1 1
  spline S72 degree 3 poles (10.313224, -47.690708) (9.850564, -47.806594) (9.106587, -47.64913) (8.565194, -47.7314) knots 0 0 0 0 1 1 1 1
  spline S73 degree 3 poles (8.565194, -47.7314) (7.831837, -47.842864) (7.045399, -48.036599) (6.371312, -48.354181) knots 0 0 0 0 1 1 1 1
  spline S74 degree 3 poles (6.371312, -48.354181) (4.931136, -49.033576) (3.52015, -50.671027) (3.687346, -52.344746) knots 0 0 0 0 1 1 1 1
  spline S75 degree 3 poles (3.687346, -52.344746) (3.84923, -53.966275) (5.54595, -54.936715) (6.952514, -55.34895) knots 0 0 0 0 1 1 1 1
  spline S76 degree 3 poles (6.952514, -55.34895) (8.360844, -55.762959) (9.660366, -55.97527) (11.127085, -56.100003) knots 0 0 0 0 1 1 1 1
  spline S77 degree 3 poles (11.127085, -56.100003) (13.05027, -56.264543) (14.527604, -56.046039) (16.420715, -56.751975) knots 0 0 0 0 1 1 1 1
  spline S78 degree 3 poles (16.420715, -56.751975) (17.989162, -57.336714) (19.439953, -58.182421) (20.717359, -59.26521) knots 0 0 0 0 1 1 1 1
  spline S79 degree 3 poles (20.717359, -59.26521) (21.727611, -60.121531) (22.561817, -61.252089) (23.714487, -61.929716) knots 0 0 0 0 1 1 1 1
  spline S80 degree 3 poles (23.714487, -61.929716) (24.597352, -62.448109) (25.696946, -62.677228) (26.697463, -62.838232) knots 0 0 0 0 1 1 1 1
  spline S81 degree 3 poles (26.697463, -62.838232) (27.565285, -62.978002) (28.406569, -62.789577) (29.262891, -62.682536) knots 0 0 0 0 1 1 1 1
  spline S82 degree 3 poles (29.262891, -62.682536) (29.95998, -62.595842) (30.683607, -62.562226) (31.365659, -62.375569) knots 0 0 0 0 1 1 1 1
  spline S83 degree 3 poles (31.365659, -62.375569) (33.212762, -61.869562) (34.995294, -60.650541) (36.329318, -59.294402) knots 0 0 0 0 1 1 1 1
  spline S84 degree 3 poles (36.329318, -59.294402) (36.767208, -58.849433) (37.060906, -58.270884) (37.30418, -57.702067) knots 0 0 0 0 1 1 1 1
  spline S85 degree 3 poles (37.30418, -57.702067) (37.442182, -57.376524) (37.510297, -57.017364) (37.83938, -56.825398) knots 0 0 0 0 1 1 1 1
  spline S86 degree 3 poles (37.83938, -56.825398) (38.025153, -56.718359) (38.238349, -56.697128) (38.436505, -56.62282) knots 0 0 0 0 1 1 1 1
  spline S87 degree 3 poles (38.436505, -56.62282) (39.124747, -56.362738) (39.833337, -56.089388) (40.491502, -55.762074) knots 0 0 0 0 1 1 1 1
  spline S88 degree 3 poles (40.491502, -55.762074) (41.118705, -55.449799) (41.732638, -55.089754) (42.377535, -54.815518) knots 0 0 0 0 1 1 1 1
  spline S89 degree 3 poles (42.377535, -54.815518) (43.043661, -54.530667) (43.728364, -54.297126) (44.391837, -54.000774) knots 0 0 0 0 1 1 1 1
  spline S90 degree 3 poles (44.391837, -54.000774) (45.707282, -53.412496) (46.989113, -52.748138) (48.310748, -52.172245) knots 0 0 0 0 1 1 1 1
  spline S91 degree 3 poles (48.310748, -52.172245) (49.548347, -51.63262) (50.784176, -51.14961) (51.992581, -50.538333) knots 0 0 0 0 1 1 1 1
  spline S92 degree 3 poles (51.992581, -50.538333) (53.409758, -49.822665) (55.098517, -49.512161) (56.341421, -48.466528) knots 0 0 0 0 1 1 1 1
  spline S93 degree 3 poles (28.978037, -60.686812) (27.383937, -60.927428) (25.770372, -60.257765) (24.651313, -59.136938) knots 0 0 0 0 1 1 1 1
  spline S94 degree 3 poles (24.651313, -59.136938) (24.171845, -58.657469) (23.390715, -57.669336) (24.265615, -57.139444) knots 0 0 0 0 1 1 1 1
  spline S95 degree 3 poles (24.265615, -57.139444) (24.956511, -56.721012) (25.336016, -57.450832) (25.740292, -57.870146) knots 0 0 0 0 1 1 1 1
  spline S96 degree 3 poles (25.740292, -57.870146) (26.355112, -58.505313) (27.211433, -59.013975) (28.111986, -59.043167) knots 0 0 0 0 1 1 1 1
  spline S97 degree 3 poles (28.111986, -59.043167) (30.511103, -59.122783) (32.145018, -57.081058) (32.97303, -55.048176) knots 0 0 0 0 1 1 1 1
  spline S98 degree 3 poles (32.97303, -55.048176) (33.161457, -54.587285) (33.397652, -54.149392) (33.519731, -53.662845) knots 0 0 0 0 1 1 1 1
  spline S99 degree 3 poles (33.519731, -53.662845) (33.678078, -53.027681) (33.766541, -52.389863) (33.83643, -51.73966) knots 0 0 0 0 1 1 1 1
  spline S100 degree 3 poles (33.83643, -51.73966) (33.89835, -51.156689) (34.002741, -50.558678) (33.969125, -49.970399) knots 0 0 0 0 1 1 1 1
  spline S101 degree 3 poles (33.969125, -49.970399) (33.835545, -47.671246) (32.848295, -43.802757) (30.301446, -43.052589) knots 0 0 0 0 1 1 1 1
  spline S102 degree 3 poles (30.301446, -43.052589) (29.713165, -42.879202) (29.156734, -42.894242) (28.554301, -42.929627) knots 0 0 0 0 1 1 1 1
  spline S103 degree 3 poles (28.554301, -42.929627) (27.957176, -42.964126) (27.370665, -43.076476) (26.825736, -43.334787) knots 0 0 0 0 1 1 1 1
  spline S104 degree 3 poles (26.825736, -43.334787) (26.375456, -43.547983) (25.659793, -44.249494) (25.465174, -44.713042) knots 0 0 0 0 1 1 1 1
  spline S105 degree 3 poles (25.465174, -44.713042) (25.208629, -45.323436) (25.303285, -46.625612) (24.171845, -46.255837) knots 0 0 0 0 1 1 1 1
  spline S106 degree 3 poles (24.171845, -46.255837) (23.004132, -45.874562) (23.952453, -43.923951) (24.425733, -43.318864) knots 0 0 0 0 1 1 1 1
  spline S107 degree 3 poles (24.425733, -43.318864) (25.822562, -41.533681) (27.41136, -41.177175) (29.615857, -41.251483) knots 0 0 0 0 1 1 1 1
  spline S108 degree 3 poles (29.615857, -41.251483) (31.779665, -41.324024) (33.483458, -43.05436) (34.390204, -44.886429) knots 0 0 0 0 1 1 1 1
  spline S109 degree 3 poles (34.390204, -44.886429) (34.65825, -45.427822) (34.820139, -46.016101) (34.994408, -46.59111) knots 0 0 0 0 1 1 1 1
  spline S110 degree 3 poles (34.994408, -46.59111) (35.265105, -47.486358) (35.486263, -48.417874) (35.576497, -49.351158) knots 0 0 0 0 1 1 1 1
  spline S111 degree 3 poles (35.576497, -49.351158) (35.656113, -50.172095) (35.600381, -51.013379) (35.502188, -51.828123) knots 0 0 0 0 1 1 1 1
  spline S112 degree 3 poles (35.502188, -51.828123) (35.4093, -52.600406) (35.313761, -53.358532) (35.121795, -54.114007) knots 0 0 0 0 1 1 1 1
  spline S113 degree 3 poles (35.121795, -54.114007) (34.997065, -54.603207) (34.772365, -55.049947) (34.579517, -55.512607) knots 0 0 0 0 1 1 1 1
  spline S114 degree 3 poles (34.579517, -55.512607) (33.540076, -58.00638) (31.815933, -60.259534) (28.978037, -60.686812) knots 0 0 0 0 1 1 1 1
  spline S115 degree 3 poles (19.265683, -53.370033) (19.167491, -52.708331) (19.070178, -52.047512) (18.971985, -51.385808) knots 0 0 0 0 1 1 1 1
  spline S116 degree 3 poles (18.971985, -51.385808) (18.419977, -51.35573) (17.868854, -51.459231) (17.319497, -51.510541) knots 0 0 0 0 1 1 1 1
  spline S117 degree 3 poles (17.319497, -51.510541) (16.495021, -51.587503) (15.667008, -51.623773) (14.842532, -51.69985) knots 0 0 0 0 1 1 1 1
  spline S118 degree 3 poles (14.842532, -51.69985) (14.245406, -51.753814) (13.474892, -51.880316) (13.428009, -51.005418) knots 0 0 0 0 1 1 1 1
  spline S119 degree 3 poles (13.428009, -51.005418) (13.38997, -50.298596) (14.136599, -50.241981) (14.626682, -50.149979) knots 0 0 0 0 1 1 1 1
  spline S120 degree 3 poles (14.626682, -50.149979) (15.159231, -50.050901) (15.717433, -50.053555) (16.25794, -50.005784) knots 0 0 0 0 1 1 1 1
  spline S121 degree 3 poles (16.25794, -50.005784) (17.156722, -49.927053) (18.052853, -49.841244) (18.953406, -49.793473) knots 0 0 0 0 1 1 1 1
  spline S122 degree 3 poles (18.953406, -49.793473) (19.056912, -48.779687) (19.161298, -47.766785) (19.265683, -46.752999) knots 0 0 0 0 1 1 1 1
  spline S123 degree 3 poles (19.265683, -46.752999) (17.767119, -47.627014) (16.233168, -48.298448) (14.615181, -48.905303) knots 0 0 0 0 1 1 1 1
  spline S124 degree 3 poles (14.615181, -48.905303) (13.983554, -49.142386) (13.374928, -49.407776) (12.715883, -49.564354) knots 0 0 0 0 1 1 1 1
  spline S125 degree 3 poles (12.715883, -49.564354) (12.015252, -49.730665) (10.570654, -50.281788) (10.330032, -49.222003) knots 0 0 0 0 1 1 1 1
  spline S126 degree 3 poles (10.330032, -49.222003) (10.074373, -48.094099) (11.882557, -48.112675) (12.564609, -47.918056) knots 0 0 0 0 1 1 1 1
  spline S127 degree 3 poles (12.564609, -47.918056) (13.144926, -47.751748) (13.677475, -47.488127) (14.248943, -47.305008) knots 0 0 0 0 1 1 1 1
  spline S128 degree 3 poles (14.248943, -47.305008) (16.010245, -46.740613) (17.766234, -45.878099) (19.282491, -44.810352) knots 0 0 0 0 1 1 1 1
  spline S129 degree 3 poles (19.282491, -44.810352) (19.838036, -44.419344) (20.813786, -43.295863) (21.375524, -44.369805) knots 0 0 0 0 1 1 1 1
  spline S130 degree 3 poles (21.375524, -44.369805) (21.623225, -44.843966) (21.205677, -45.748943) (21.074753, -46.255837) knots 0 0 0 0 1 1 1 1
  spline S131 degree 3 poles (21.074753, -46.255837) (20.722667, -47.619936) (20.597936, -49.09373) (20.582899, -50.501177) knots 0 0 0 0 1 1 1 1
  spline S132 degree 3 poles (20.582899, -50.501177) (20.571398, -51.667119) (20.79167, -52.910909) (21.075639, -54.039698) knots 0 0 0 0 1 1 1 1
  spline S133 degree 3 poles (21.075639, -54.039698) (21.198598, -54.529784) (21.40649, -55.096833) (20.89252, -55.44626) knots 0 0 0 0 1 1 1 1
  spline S134 degree 3 poles (20.89252, -55.44626) (20.396243, -55.783304) (20.060965, -55.410875) (19.609806, -55.24545) knots 0 0 0 0 1 1 1 1
  spline S135 degree 3 poles (19.609806, -55.24545) (19.296643, -55.131332) (18.966678, -55.051716) (18.644671, -54.967675) knots 0 0 0 0 1 1 1 1
  spline S136 degree 3 poles (18.644671, -54.967675) (16.917876, -54.516515) (14.394024, -54.225471) (12.62742, -54.410359) knots 0 0 0 0 1 1 1 1
  spline S137 degree 3 poles (12.62742, -54.410359) (12.017023, -54.474052) (10.930699, -54.677516) (10.608693, -53.979544) knots 0 0 0 0 1 1 1 1
  spline S138 degree 3 poles (10.608693, -53.979544) (10.519344, -53.784924) (10.514922, -53.552266) (10.574191, -53.348802) knots 0 0 0 0 1 1 1 1
  spline S139 degree 3 poles (10.574191, -53.348802) (10.803312, -52.571212) (11.94006, -52.759638) (12.542493, -52.723368) knots 0 0 0 0 1 1 1 1
  spline S140 degree 3 poles (12.542493, -52.723368) (14.210019, -52.62429) (15.850127, -52.776446) (17.495537, -53.030335) knots 0 0 0 0 1 1 1 1
  spline S141 degree 3 poles (17.495537, -53.030335) (18.088241, -53.122337) (18.672094, -53.305456) (19.265683, -53.370033) knots 0 0 0 0 1 1 1 1
  spline S142 degree 3 poles (40.06511, -52.62429) (40.860392, -52.591559) (41.59729, -52.075818) (42.294379, -51.729044) knots 0 0 0 0 1 1 1 1
  spline S143 degree 3 poles (42.294379, -51.729044) (42.795963, -51.478693) (43.328512, -51.294691) (43.831867, -51.047878) knots 0 0 0 0 1 1 1 1
  spline S144 degree 3 poles (43.831867, -51.047878) (44.770459, -50.586986) (45.85767, -49.923514) (46.740529, -49.357351) knots 0 0 0 0 1 1 1 1
  spline S145 degree 3 poles (46.740529, -49.357351) (47.266, -49.02119) (48.26917, -48.614262) (48.596484, -48.112675) knots 0 0 0 0 1 1 1 1
  spline S146 degree 3 poles (48.596484, -48.112675) (46.575104, -46.089526) (44.574956, -44.96693) (41.845871, -44.147762) knots 0 0 0 0 1 1 1 1
  spline S147 degree 3 poles (41.845871, -44.147762) (40.905509, -43.865565) (39.843067, -43.444483) (38.848743, -43.601061) knots 0 0 0 0 1 1 1 1
  spline S148 degree 3 poles (38.848743, -43.601061) (39.057517, -44.616618) (39.161903, -45.588825) (39.258327, -46.62119) knots 0 0 0 0 1 1 1 1
  spline S149 degree 3 poles (39.258327, -46.62119) (39.848377, -46.698153) (40.732122, -46.376146) (41.080666, -47.04139) knots 0 0 0 0 1 1 1 1
  spline S150 degree 3 poles (41.080666, -47.04139) (41.188591, -47.248393) (41.203629, -47.509357) (41.125781, -47.7314) knots 0 0 0 0 1 1 1 1
  spline S151 degree 3 poles (41.125781, -47.7314) (41.04705, -47.95698) (40.792276, -48.161329) (40.564925, -48.216178) knots 0 0 0 0 1 1 1 1
  spline S152 degree 3 poles (40.564925, -48.216178) (40.17746, -48.310832) (38.600162, -48.392219) (38.221541, -48.299331) knots 0 0 0 0 1 1 1 1
  spline S153 degree 3 poles (38.221541, -48.299331) (37.796919, -48.194945) (37.616454, -47.80394) (37.612032, -47.404971) knots 0 0 0 0 1 1 1 1
  spline S154 degree 3 poles (37.612032, -47.404971) (37.600531, -46.272646) (37.574876, -45.148279) (37.249333, -44.053106) knots 0 0 0 0 1 1 1 1
  spline S155 degree 3 poles (37.249333, -44.053106) (37.113099, -43.593985) (36.854786, -43.216246) (36.672552, -42.781893) knots 0 0 0 0 1 1 1 1
  spline S156 degree 3 poles (36.672552, -42.781893) (36.519513, -42.420079) (36.577013, -41.982189) (36.916711, -41.745991) knots 0 0 0 0 1 1 1 1
  spline S157 degree 3 poles (36.916711, -41.745991) (37.200677, -41.548718) (37.6023, -41.577027) (37.931382, -41.588527) knots 0 0 0 0 1 1 1 1
  spline S158 degree 3 poles (37.931382, -41.588527) (38.762934, -41.616836) (39.609526, -41.743338) (40.412769, -41.952994) knots 0 0 0 0 1 1 1 1
  spline S159 degree 3 poles (40.412769, -41.952994) (41.02228, -42.111344) (41.595522, -42.373194) (42.197955, -42.557198) knots 0 0 0 0 1 1 1 1
  spline S160 degree 3 poles (42.197955, -42.557198) (43.849558, -43.060553) (45.497625, -43.659447) (46.935149, -44.638733) knots 0 0 0 0 1 1 1 1
  spline S161 degree 3 poles (46.935149, -44.638733) (47.440272, -44.982853) (47.902935, -45.382708) (48.386828, -45.756019) knots 0 0 0 0 1 1 1 1
  spline S162 degree 3 poles (48.386828, -45.756019) (48.987492, -46.218682) (50.471902, -47.416472) (50.536478, -48.201139) knots 0 0 0 0 1 1 1 1
  spline S163 degree 3 poles (50.536478, -48.201139) (50.605479, -49.038884) (48.823835, -49.989861) (48.191325, -50.367597) knots 0 0 0 0 1 1 1 1
  spline S164 degree 3 poles (48.191325, -50.367597) (47.316424, -50.889531) (46.451256, -51.398194) (45.558664, -51.891816) knots 0 0 0 0 1 1 1 1
  spline S165 degree 3 poles (45.558664, -51.891816) (45.199505, -52.090858) (44.867768, -52.334131) (44.496223, -52.511943) knots 0 0 0 0 1 1 1 1